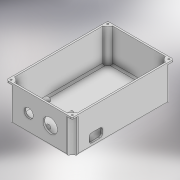
# Autodesk Inventor part: Chasis Raspberry Pi
Saved by Autodesk Inventor 2021.4 (Build 254397000, 397)
## iProperties
Created: 2022-12-12
Part Number: Chasis Raspberry Pi
Material: Genérico
Document SubType Name: Modeling
Designer: crist
Density: 1 g/cm^3
Appearance: Valor por defecto
Mass: 48.8958 g
Surface Area: 495.771 cm^2
Volume: 48.8958 cm^3
Author: crist
Autodesk Inventor part; units mm, degrees
ref_plane "YZ Plane" through (0, 0, 0) normal (1, 0, 0) x (0, 1, 0)
ref_plane "XZ Plane" through (0, 0, 0) normal (0, 1, 0) x (-1, 0, 0)
ref_plane "XY Plane" through (0, 0, 0) normal (0, 0, 1) x (1, 0, 0)
sketch "Boceto1" plane through (0, 0, 0) normal (0, 1, 0) x (-1, 0, 0)
  line L0 (0, 0) -> (78, 0)
  line L1 (78, 0) -> (78, -120)
  line L2 (78, -120) -> (0, -120)
  line L3 (0, -120) -> (0, 0)
  dimension "d0" = 78
  dimension "d1" = 120
  constraints: 8 end point, 2 parallel, 1 horizontal, 1 perpendicular
  measures "d0" distance of L1.end L2.end
  measures "d1" distance of L0.end L1.end
extrude "Extrusión1" add sketch "Boceto1" along normal blind 2
sketch "Boceto2" plane through (0, 2, 0) normal (0, 1, 0) x (1, 0, 0)
  line L0 (0, 120) -> (0, 0) projected
  line L1 (0, 0) -> (-78, 0) projected
  line L2 (-78, 0) -> (-78, 120) projected
  line L3 (-78, 120) -> (0, 120) projected
  line L4 (-76, 118) -> (-76, 2)
  line L5 (-76, 2) -> (-2, 2)
  line L6 (-2, 2) -> (-2, 118)
  line L7 (-2, 118) -> (-76, 118)
  dimension "d4" = 2
  constraints: 8 end point, 3 other
  measures "d4" distance between parallel lines of L2 L4
extrude "Extrusión2" add sketch "Boceto2" along normal blind 40
sketch "Boceto3" plane through (-78, 0, 0) normal (0, 0, 1) x (1, 0, 0)
  line L0 (0, 42) -> (78, 42) projected
  line L1 (78, 42) -> (78, 21)
  line L2 (78, 0) -> (78, 42) projected
  line L3 (78, 21) -> (68, 21)
  line L4 (68, 21) -> (68, 37)
  line L5 (68, 37) -> (36, 37)
  line L6 (36, 37) -> (36, 5)
  line L7 (36, 5) -> (68, 5)
  line L8 (68, 5) -> (68, 21)
  line L9 (36, 37) -> (38, 37)
  line L10 (38, 37) -> (38, 35)
  circle A0 centre (38, 35) radius 1
  line L11 (52, 37) -> (52, 25.2486)
  line L12 (36, 21) -> (50.0571, 21)
  circle A1 centre (66, 35) radius 1
  circle A2 centre (38, 7) radius 1
  circle A3 centre (66, 7) radius 1
  dimension "d7" = 21
  dimension "d8" = 10
  dimension "d9" = 16
  dimension "d10" = 32
  dimension "d11" = 32
  dimension "d12" = 32
  dimension "d13" = 2
  dimension "d14" = 2
  dimension "d15" = 2
  constraints: 22 end point, 5 perpendicular, 4 centre point, 3 midpoint, 3 symmetric about line, 2 point on line, 1 coincident, 1 horizontal, 1 vertical, 3 other
  measures "d7" distance of L0.end L1.end
  measures "d8" distance of L1.end L3.end
  measures "d9" distance of L3.end L4.end
  measures "d10" distance of L4.end L5.end
  measures "d11" distance of L5.end L6.end
  measures "d12" distance of L6.end L7.end
  measures "d13" distance of L5.end L9.end
  measures "d14" distance of L9.end L10.end
  measures "d15" diameter of A0
extrude "Extrusión3" cut sketch "Boceto3" against normal blind 2 contours A0 | A1 | A2 | A3
sketch "Boceto4" plane through (-78, 0, 0) normal (0, 0, 1) x (1, 0, 0)
  line L0 (0, 0) -> (0, 42) projected
  line L1 (0, 42) -> (0, 21)
  line L2 (0, 0) -> (78, 0) projected
  line L3 (0, 21) -> (5, 21)
  line L4 (5, 21) -> (5, 29.01)
  line L5 (5, 29.01) -> (33.28, 29.01)
  line L6 (33.28, 29.01) -> (33.28, 12.99)
  line L7 (33.28, 12.99) -> (5, 12.99)
  line L8 (5, 12.99) -> (5, 21)
  line L9 (5, 21) -> (33.28, 21)
  line L10 (33.28, 21) -> (26.425, 21)
  circle A0 centre (26.425, 21) radius 5.5
  line L11 (33.28, 29.01) -> (31.44, 29.01)
  line L12 (31.44, 29.01) -> (31.44, 27.05)
  circle A1 centre (31.44, 27.05) radius 1
  circle A2 centre (31.44, 14.95) radius 1
  dimension "d18" = 21
  dimension "d19" = 8.01
  dimension "d20" = 28.28
  dimension "d21" = 16.02
  dimension "d22" = 28.28
  dimension "d23" = 6.855
  dimension "d24" = 11
  dimension "d25" = 1.84
  dimension "d26" = 1.96
  dimension "d27" = 2
  dimension "d104" = 5
  constraints: 22 end point, 6 perpendicular, 3 centre point, 2 coincident, 2 point on line, 1 horizontal, 1 midpoint, 1 symmetric about line, 1 other
  measures "d18" distance of L0.end L1.end
  measures "d19" distance of L3.end L4.end
  measures "d20" distance of L4.end L5.end
  measures "d21" distance of L5.end L6.end
  measures "d22" distance of L6.end L7.end
  measures "d23" distance of L9.end L10.end
  measures "d24" diameter of A0
  measures "d25" distance of L5.end L11.end
  measures "d26" distance of L11.end L12.end
  measures "d27" diameter of A1
  measures "d104" distance of L1.end L3.end
extrude "Extrusión4" cut sketch "Boceto4" against normal blind 2 contours A0 L9 | L9 A0 | A1 | A2
fillet "Empalme1" radius 2 16 edges at (-76, 2, -60) (0, 21, 0) (-78, 21, 0) (-39, 0, 0) (0, 0, -60) (-39, 2, -118) (-76, 22, -118) (0, 21, -120) (-2, 22, -118) (-2, 22, -2) (-78, 21, -120) (-2, 2, -60) (-76, 22, -2) (-39, 2, -2) (-39, 0, -120) (-78, 0, -60)
sketch "Boceto5" plane through (-4, 42, -2) normal (0, 0, -1) x (-1, 0, 0)
  line L0 (72, -42) -> (-2, -42) projected
  arc A0 (-4, -40) -> (-2, -42) centre (-2, -40) ccw projected
  line L1 (-4, -40) -> (-4, 0) projected
  line L2 (-4, 0) -> (0, 0) projected
  line L3 (0, 0) -> (70, 0) projected
  line L4 (70, 0) -> (74, 0) projected
  line L5 (74, 0) -> (74, -40) projected
  line L6 (0, 0) -> (0, -38) projected
  line L7 (0, -38) -> (70, -38) projected
  line L8 (70, 0) -> (70, -38) projected
  circle A1 centre (42.56, -27.05) radius 1 projected
  circle A2 centre (42.56, -14.95) radius 1 projected
  circle A3 centre (47.575, -21) radius 5.5 projected
  circle A4 centre (36, -35) radius 1 projected
  circle A5 centre (36, -7) radius 1 projected
  circle A6 centre (8, -35) radius 1 projected
  circle A7 centre (8, -7) radius 1 projected
  circle A8 centre (8, -7) radius 2.5
  circle A9 centre (36, -7) radius 2.5
  circle A10 centre (36, -35) radius 2.5
  circle A11 centre (8, -35) radius 2.5
  arc A12 (72, -42) -> (74, -40) centre (72, -40) ccw projected
  point P0 (-4, -42)
  dimension "d31" = 1.5
  dimension "d32" = 1.5
  dimension "d33" = 1.5
  dimension "d35" = 1.5
  constraints: 4 centre point
  measures "d31" radial gap between concentric circles of A7 A8
  measures "d32" radial gap between concentric circles of A5 A9
  measures "d33" radial gap between concentric circles of A4 A10
  measures "d35" radial gap between concentric circles of A6 A11
extrude "Extrusión5" add sketch "Boceto5" along normal blind 10 contours A8 | A9 | A10 | A11
sketch "Boceto6" plane through (-4, 42, -2) normal (0, 0, -1) x (-1, 0, 0)
  circle A0 centre (8, -7) radius 1 projected
  circle A1 centre (36, -7) radius 1 projected
  line L0 (8, -7) -> (36, -7)
  line L1 (22, -7) -> (22, -21)
  circle A2 centre (22, -21) radius 8.5
  point P0 (-4, -42)
  dimension "d38" = 14
  dimension "d39" = 17
  constraints: 4 end point, 1 centre point, 1 coincident, 1 horizontal, 1 midpoint, 1 vertical
  measures "d38" distance of L1.start L1.end
  measures "d39" diameter of A2
extrude "Extrusión6" cut sketch "Boceto6" against normal blind 2 contours A2
sketch "Boceto7" plane through (-4, 42, -2) normal (0, 0, -1) x (-1, 0, 0)
  circle A0 centre (22, -21) radius 8.5 projected
  circle A1 centre (8, -7) radius 2.5 projected
  circle A2 centre (36, -35) radius 2.5 projected
  circle A3 centre (8, -35) radius 2.5 projected
  circle A4 centre (36, -7) radius 2.5 projected
  line L0 (72, -42) -> (-2, -42) projected
  arc A5 (-4, -40) -> (-2, -42) centre (-2, -40) ccw projected
  line L1 (-4, -40) -> (-4, 0) projected
  line L2 (-4, 0) -> (0, 0) projected
  line L3 (0, 0) -> (70, 0) projected
  line L4 (70, 0) -> (74, 0) projected
  line L5 (74, 0) -> (74, -40) projected
  line L6 (0, 0) -> (0, -38) projected
  line L7 (0, -38) -> (70, -38) projected
  line L8 (70, 0) -> (70, -38) projected
  circle A6 centre (42.56, -27.05) radius 1 projected
  circle A7 centre (42.56, -14.95) radius 1 projected
  circle A8 centre (47.575, -21) radius 5.5 projected
  circle A9 centre (36, -35) radius 1 projected
  circle A10 centre (36, -7) radius 1 projected
  circle A11 centre (8, -35) radius 1 projected
  circle A12 centre (8, -7) radius 1 projected
  arc A13 (44.6263, -16.3572) -> (43.5596, -17.2415) centre (42.56, -14.95) ccw
  arc A14 (43.5596, -24.7585) -> (44.6263, -25.6428) centre (42.56, -27.05) ccw
  arc A15 (72, -42) -> (74, -40) centre (72, -40) ccw projected
  point P0 (-4, -42)
  dimension "d42" = 1.5
  dimension "d43" = 1.5
  constraints: 8 point on circle, 2 centre point
  measures "d42" radial gap between concentric circles of A7 A13
  measures "d43" radial gap between concentric circles of A6 A14
extrude "Extrusión7" add sketch "Boceto7" along normal blind 6 contours A8 A13 | A14 A8
sketch "Boceto8" plane through (-76, 42, 0) normal (0, 0, 1) x (1, 0, 0)
  line L0 (72, -38) -> (2, -38) projected
  line L1 (59.0515, -3.7406) -> (69.5704, -3.7406)
  line L2 (69.5704, -3.7406) -> (69.5704, -38)
  line L3 (69.5704, -38) -> (59.0515, -38)
  line L4 (59.0515, -38) -> (59.0515, -3.7406)
  line L5 (41.825, -36.9742) -> (28.325, -36.9742)
  line L6 (28.325, -36.9742) -> (28.325, -25.9742)
  line L7 (28.325, -25.9742) -> (41.825, -25.9742)
  line L8 (41.825, -25.9742) -> (41.825, -36.9742)
  line L9 (28.325, -16.6878) -> (38.9625, -16.6878)
  line L10 (38.9625, -16.6878) -> (38.9625, -3.7406)
  line L11 (38.9625, -3.7406) -> (28.325, -3.7406)
  line L12 (28.325, -3.7406) -> (28.325, -16.6878)
  dimension "d107" = 11
  dimension "d108" = 13.5
  constraints: 24 end point, 6 parallel, 3 horizontal, 3 perpendicular, 1 point on line
  measures "d107" distance of L7.end L5.start
  measures "d108" distance of L6.end L7.end
extrude "Extrusión8" add sketch "Boceto8" against normal blind 2
sketch "Boceto9" plane through (0, 2, -118) normal (1, 0, 0) x (0, 0, -1)
  line L0 (-85.12, 2.85) -> (-95.02, 2.85)
  line L1 (-98.02, 5.85) -> (-98.02, 10.35)
  line L2 (-95.02, 13.35) -> (-85.12, 13.35)
  line L3 (-82.12, 10.35) -> (-82.12, 5.85)
  arc A0 (-82.12, 10.35) -> (-85.12, 13.35) centre (-85.12, 10.35) ccw
  arc A1 (-85.12, 2.85) -> (-82.12, 5.85) centre (-85.12, 5.85) ccw
  arc A2 (-98.02, 5.85) -> (-95.02, 2.85) centre (-95.02, 5.85) ccw
  arc A3 (-95.02, 13.35) -> (-98.02, 10.35) centre (-95.02, 10.35) ccw
  point P0 (-118, -2)
  point P1 (0, 0)
  point P2 (-98.02, 2.85)
  point P3 (-98.02, 13.35)
  point P4 (-82.12, 13.35)
  dimension "d53" = 10.5
  dimension "d54" = 15.9
  dimension "d55" = 3
  constraints: 8 end point, 8 point on circle, 8 tangent, 6 point on line, 4 centre point, 3 equal radius, 1 horizontal, 1 perpendicular, 1 vertical
  measures "d53" distance of point (-98.02, 2.85) point (-98.02, 13.35)
  measures "d54" distance of point (-98.02, 13.35) point (-82.12, 13.35)
  measures "d55" radius of A0
extrude "Extrusión9" cut sketch "Boceto9" against normal blind 2
sketch "Boceto14" plane through (0, 0, 0) normal (0, -1, 0) x (1, 0, 0)
  arc A0 (-0.8571, -114.0615) -> (-5.9385, -119.1429) centre (0, -120) ccw
  line L0 (0, -120) -> (-2, -118)
  line L1 (-2, -118) -> (-4.2426, -115.7574)
  circle A1 centre (-4.2426, -115.7574) radius 1
  line L2 (-2, -118) -> (-76, -118) projected
  line L3 (-76, -118) -> (-76, -2) projected
  line L4 (-76, -2) -> (-2, -2) projected
  line L5 (-2, -2) -> (-2, -118) projected
  line L6 (-76, -120) -> (-2, -120) projected
  line L7 (-2, -120) -> (-76, -120) projected
  line L8 (-6.9282, -120) -> (-9.9689, -120)
  line L9 (0, -118) -> (0, -2) projected
  line L10 (0, -2) -> (0, -118) projected
  line L11 (0, -113.0718) -> (0, -112.4163)
  arc A2 (-6.9282, -120) -> (-5.9385, -119.1429) centre (-6.9282, -119) ccw
  arc A3 (-0.8571, -114.0615) -> (0, -113.0718) centre (-1, -113.0718) ccw
  arc A4 (-2, -120) -> (0, -118) centre (-2, -118) ccw projected
  line L12 (-39, -120) -> (-39, -100.8346)
  arc A5 (-72.0615, -119.1429) -> (-77.1429, -114.0615) centre (-78, -120) ccw
  line L13 (-78, -120) -> (-76, -118)
  line L14 (-76, -118) -> (-73.7574, -115.7574)
  circle A6 centre (-73.7574, -115.7574) radius 1
  line L15 (-71.0718, -120) -> (-68.0311, -120)
  line L16 (-78, -113.0718) -> (-78, -112.4163)
  arc A7 (-72.0615, -119.1429) -> (-71.0718, -120) centre (-71.0718, -119) ccw
  arc A8 (-78, -113.0718) -> (-77.1429, -114.0615) centre (-77, -113.0718) ccw
  arc A9 (-78, -118) -> (-76, -120) centre (-76, -118) ccw
  line L17 (-78, -2) -> (-78, -118) projected
  line L18 (-78, -118) -> (-78, -2) projected
  line L19 (-78, -60) -> (-55.773, -60)
  line L20 (-2, 0) -> (-76, 0) projected
  line L21 (-78, 0) -> (-76, -2)
  arc A10 (-76, 0) -> (-78, -2) centre (-76, -2) ccw
  circle A11 centre (-73.7574, -4.2426) radius 1
  arc A12 (-77.1429, -5.9385) -> (-72.0615, -0.8571) centre (-78, 0) ccw
  line L22 (-76, -2) -> (-73.7574, -4.2426)
  arc A13 (-71.0718, 0) -> (-72.0615, -0.8571) centre (-71.0718, -1) ccw
  arc A14 (-77.1429, -5.9385) -> (-78, -6.9282) centre (-77, -6.9282) ccw
  line L23 (-78, -6.9282) -> (-78, -7.5837)
  line L24 (-71.0718, 0) -> (-68.0311, 0)
  arc A15 (-5.9385, -0.8571) -> (-0.8571, -5.9385) centre (0, 0) ccw
  line L25 (0, 0) -> (-2, -2)
  line L26 (-2, -2) -> (-4.2426, -4.2426)
  circle A16 centre (-4.2426, -4.2426) radius 1
  line L27 (-6.9282, 0) -> (-9.9689, 0)
  line L28 (0, -6.9282) -> (0, -7.5837)
  arc A17 (-5.9385, -0.8571) -> (-6.9282, 0) centre (-6.9282, -1) ccw
  arc A18 (0, -6.9282) -> (-0.8571, -5.9385) centre (-1, -6.9282) ccw
  arc A19 (0, -2) -> (-2, 0) centre (-2, -2) ccw
  point P0 (0, 0)
  point P1 (-6, -120)
  point P2 (0, -114)
  point P3 (-72, -120)
  point P4 (-78, -114)
  point P5 (-76, -2)
  point P6 (-72, 0)
  point P7 (-78, -6)
  point P8 (-6, 0)
  point P9 (0, -6)
  dimension "d88" = 12
  dimension "d89" = 2
  dimension "d90" = 1
  constraints: 50 symmetric about line, 42 point on circle, 36 end point, 19 centre point, 12 point on line, 4 coincident, 4 tangent, 2 midpoint, 1 equal radius, 1 horizontal, 1 vertical, 15 other
  measures "d88" diameter of A0
  measures "d89" diameter of A1
  measures "d90" radius of A2
extrude "Extrusión10" cut sketch "Boceto14" against normal blind 42 contours A3 L9 A4 L0 L5 A0 | L5 L1 A1 A0 | A1 L1 A0 | A15 A16 L26 L5 | L5 L25 A19 L9 A18 A15 | L2 A0 A1 L1 | L0 A4 L6 A2 A0 L2 | L1 A1 A0 | L26 A16 A15 L4 | L4 A15 A17 L20 A19 L25 | A15 L26 A16 | L26 A15 A16 | A12 A11 L22 L4 | L4 L21 A10 L20 A13 A12 | A5 A7 L6 A9 L13 L2 | L2 L14 A6 A5 | L22 A11 A12 L3 | L3 A12 A14 L17 A10 L21 | A12 L22 A11 | L13 A9 L17 A8 A5 L3 | L3 A5 A6 L14 | A6 L14 A5 | L22 A12 A11 | A6 A5 L14
sketch "Boceto16" plane through (0, 2, 0) normal (0, 1, 0) x (1, 0, 0)
  line L0 (-71.0718, 120) -> (-6.9282, 120) projected
  arc A0 (-5.9385, 119.1429) -> (-6.9282, 120) centre (-6.9282, 119) ccw projected
  arc A1 (-5.9385, 119.1429) -> (-4.4721, 116) centre (0, 120) ccw projected
  arc A2 (-4.4721, 116) -> (-4, 115.5279) centre (0, 120) ccw projected
  arc A3 (-4, 115.5279) -> (-0.8571, 114.0615) centre (0, 120) ccw projected
  arc A4 (0, 113.0718) -> (-0.8571, 114.0615) centre (-1, 113.0718) ccw projected
  line L1 (0, 113.0718) -> (0, 6.9282) projected
  line L2 (-6.9282, 0) -> (-71.0718, 0) projected
  line L3 (-73.5279, 116) -> (-4.4721, 116) projected
  line L4 (-4.4721, 4) -> (-73.5279, 4) projected
  line L5 (-4, 115.5279) -> (-4, 4.4721) projected
  arc A5 (-8, 120) -> (-5.9628, 114.6667) centre (0, 120) ccw
  line L6 (-7.746, 118) -> (-76, 118)
  line L7 (-76, 118) -> (-76, 2)
  line L8 (-76, 2) -> (-2, 2)
  line L9 (-2, 2) -> (-2, 112.254)
  arc A6 (-6.9282, 116) -> (0, 112) centre (0, 120) ccw
  arc A7 (-77.1429, 114.0615) -> (-74, 115.5279) centre (-78, 120) ccw projected
  arc A8 (-74, 115.5279) -> (-73.5279, 116) centre (-78, 120) ccw projected
  arc A9 (-73.5279, 116) -> (-72.0615, 119.1429) centre (-78, 120) ccw projected
  arc A10 (-71.0718, 120) -> (-72.0615, 119.1429) centre (-71.0718, 119) ccw projected
  arc A11 (-77.1429, 114.0615) -> (-78, 113.0718) centre (-77, 113.0718) ccw projected
  line L10 (-78, 6.9282) -> (-78, 113.0718) projected
  arc A12 (-78, 6.9282) -> (-77.1429, 5.9385) centre (-77, 6.9282) ccw projected
  arc A13 (-74, 4.4721) -> (-77.1429, 5.9385) centre (-78, 0) ccw projected
  arc A14 (-73.5279, 4) -> (-74, 4.4721) centre (-78, 0) ccw projected
  arc A15 (-72.0615, 0.8571) -> (-73.5279, 4) centre (-78, 0) ccw projected
  arc A16 (-72.0615, 0.8571) -> (-71.0718, 0) centre (-71.0718, 1) ccw projected
  line L11 (-74, 4.4721) -> (-74, 115.5279) projected
  line L12 (-39, 120) -> (-39, 111.48)
  line L13 (-74, 60) -> (-65.0964, 60)
  arc A17 (-71.0718, 120) -> (-72.0615, 119.1429) centre (-71.0718, 119) ccw
  arc A18 (-73.5279, 116) -> (-72.0615, 119.1429) centre (-78, 120) ccw
  arc A19 (-74, 115.5279) -> (-73.5279, 116) centre (-78, 120) ccw
  arc A20 (-77.1429, 114.0615) -> (-74, 115.5279) centre (-78, 120) ccw
  arc A21 (-77.1429, 114.0615) -> (-78, 113.0718) centre (-77, 113.0718) ccw
  arc A22 (-72.0372, 114.6667) -> (-70, 120) centre (-78, 120) ccw
  arc A23 (-78, 112) -> (-71.0718, 116) centre (-78, 120) ccw
  arc A24 (-74, 4.4721) -> (-77.1429, 5.9385) centre (-78, 0) ccw
  arc A25 (-73.5279, 4) -> (-74, 4.4721) centre (-78, 0) ccw
  arc A26 (-72.0615, 0.8571) -> (-73.5279, 4) centre (-78, 0) ccw
  arc A27 (-72.0615, 0.8571) -> (-71.0718, 0) centre (-71.0718, 1) ccw
  arc A28 (-78, 6.9282) -> (-77.1429, 5.9385) centre (-77, 6.9282) ccw
  arc A29 (-73.5279, 4) -> (-74, 4.4721) centre (-78, 0) ccw
  arc A30 (-74, 4.4721) -> (-77.1429, 5.9385) centre (-78, 0) ccw
  arc A31 (-78, 6.9282) -> (-77.1429, 5.9385) centre (-77, 6.9282) ccw
  arc A32 (-72.0615, 0.8571) -> (-71.0718, 0) centre (-71.0718, 1) ccw
  arc A33 (-70, 0) -> (-72.0372, 5.3333) centre (-78, 0) ccw
  arc A34 (-72.0615, 0.8571) -> (-73.5279, 4) centre (-78, 0) ccw
  arc A35 (-71.0718, 4) -> (-78, 8) centre (-78, 0) ccw
  arc A36 (-0.8571, 5.9385) -> (-4, 4.4721) centre (0, 0) ccw projected
  arc A37 (-4, 4.4721) -> (-4.4721, 4) centre (0, 0) ccw projected
  arc A38 (-4.4721, 4) -> (-5.9385, 0.8571) centre (0, 0) ccw projected
  arc A39 (-6.9282, 0) -> (-5.9385, 0.8571) centre (-6.9282, 1) ccw projected
  arc A40 (-0.8571, 5.9385) -> (0, 6.9282) centre (-1, 6.9282) ccw projected
  arc A41 (-0.8571, 5.9385) -> (0, 6.9282) centre (-1, 6.9282) ccw
  arc A42 (-0.8571, 5.9385) -> (-4, 4.4721) centre (0, 0) ccw
  arc A43 (-4, 4.4721) -> (-4.4721, 4) centre (0, 0) ccw
  arc A44 (-4.4721, 4) -> (-5.9385, 0.8571) centre (0, 0) ccw
  arc A45 (-6.9282, 0) -> (-5.9385, 0.8571) centre (-6.9282, 1) ccw
  arc A46 (-5.9628, 5.3333) -> (-8, 0) centre (0, 0) ccw
  arc A47 (-6.9282, 0) -> (-5.9385, 0.8571) centre (-6.9282, 1) ccw
  arc A48 (-6.9282, 0) -> (-5.9385, 0.8571) centre (-6.9282, 1) ccw
  arc A49 (-4.4721, 4) -> (-5.9385, 0.8571) centre (0, 0) ccw
  arc A50 (-4.4721, 4) -> (-5.9385, 0.8571) centre (0, 0) ccw
  arc A51 (-4, 4.4721) -> (-4.4721, 4) centre (0, 0) ccw
  arc A52 (-4, 4.4721) -> (-4.4721, 4) centre (0, 0) ccw
  arc A53 (-0.8571, 5.9385) -> (-4, 4.4721) centre (0, 0) ccw
  arc A54 (-0.8571, 5.9385) -> (-4, 4.4721) centre (0, 0) ccw
  arc A55 (0, 8) -> (-6.9282, 4) centre (0, 0) ccw
  arc A56 (-0.8571, 5.9385) -> (0, 6.9282) centre (-1, 6.9282) ccw
  arc A57 (-0.8571, 5.9385) -> (0, 6.9282) centre (-1, 6.9282) ccw
  point P0 (0, 0)
  point P1 (-70.254, 118)
  point P2 (-76, 112.254)
  point P3 (-70.254, 2)
  point P4 (-76, 7.746)
  point P5 (-72.0372, 5.3333)
  point P6 (-78, 8)
  point P7 (-78, 112)
  point P8 (-7.746, 2)
  point P9 (-2, 7.746)
  point P10 (-5.9628, 5.3333)
  point P11 (-8, 0)
  point P12 (0, 8)
  dimension "d93" = 2
  constraints: 84 point on circle, 48 symmetric about line, 38 centre point, 12 end point, 3 point on line, 2 midpoint, 1 horizontal, 1 vertical, 37 other
  measures "d93" radial gap between concentric circles of A1 A5
extrude "Extrusión11" add sketch "Boceto16" along normal blind 40 contours L0 A22 L6 A9 A10 | A22 L3 A9 L6 | L0 A0 A1 L3 A5 | A22 A23 L11 A8 L3 | A7 L11 A23 L7 | L7 A23 L10 A11 A7 | L3 A2 L5 A6 A5 | A35 L11 A13 L7 | L7 A13 A12 L10 A35 | A3 A4 L1 A6 L5 | A35 A33 L4 A14 L11 | A55 L9 A36 L5 | L5 A37 L4 A46 A55 | A55 L1 A40 A36 L9 | L4 A33 L8 A15 | L8 A33 L2 A16 A15 | A38 L8 A46 L4 | A38 A39 L2 A46 L8
sketch "Boceto17" plane through (0, 42, 0) normal (0, 1, 0) x (1, 0, 0)
  line L0 (-71.0718, 120) -> (-6.9282, 120) projected
  arc A0 (-5.9385, 119.1429) -> (-6.9282, 120) centre (-6.9282, 119) ccw projected
  arc A1 (-5.9385, 119.1429) -> (-0.8571, 114.0615) centre (0, 120) ccw projected
  arc A2 (0, 113.0718) -> (-0.8571, 114.0615) centre (-1, 113.0718) ccw projected
  line L1 (0, 113.0718) -> (0, 6.9282) projected
  line L2 (-2, 7.746) -> (-2, 112.254) projected
  arc A3 (-7.746, 118) -> (-2, 112.254) centre (0, 120) ccw projected
  line L3 (-7.746, 118) -> (-70.254, 118) projected
  line L4 (-70.254, 2) -> (-7.746, 2) projected
  line L5 (-71.0718, 120) -> (-6.9282, 120) projected
  line L6 (-6.9282, 120) -> (0, 120)
  line L7 (0, 120) -> (0, 113.0718)
  line L8 (0, 6.9282) -> (0, 113.0718) projected
  arc A4 (-72.0615, 0.8571) -> (-77.1429, 5.9385) centre (-78, 0) ccw projected
  arc A5 (-71.0718, 120) -> (-72.0615, 119.1429) centre (-71.0718, 119) ccw projected
  arc A6 (-72.0615, 0.8571) -> (-71.0718, 0) centre (-71.0718, 1) ccw projected
  arc A7 (-77.1429, 114.0615) -> (-72.0615, 119.1429) centre (-78, 120) ccw projected
  arc A8 (-78, 6.9282) -> (-77.1429, 5.9385) centre (-77, 6.9282) ccw projected
  arc A9 (-77.1429, 114.0615) -> (-78, 113.0718) centre (-77, 113.0718) ccw projected
  arc A10 (-76, 112.254) -> (-70.254, 118) centre (-78, 120) ccw projected
  line L9 (-76, 112.254) -> (-76, 7.746) projected
  arc A11 (-70.254, 2) -> (-76, 7.746) centre (-78, 0) ccw projected
  line L10 (-6.9282, 0) -> (-71.0718, 0) projected
  line L11 (-78, 6.9282) -> (-78, 113.0718) projected
  arc A12 (-71.0718, 120) -> (-72.0615, 119.1429) centre (-71.0718, 119) ccw projected
  line L12 (-78, 120) -> (-71.0718, 120)
  line L13 (-78, 0) -> (-71.0718, 0)
  line L14 (-71.0718, 0) -> (-6.9282, 0) projected
  line L15 (-78, 0) -> (-78, 6.9282)
  line L16 (-78, 120) -> (-78, 113.0718)
  line L17 (-78, 113.0718) -> (-78, 6.9282) projected
  arc A13 (-0.8571, 5.9385) -> (0, 6.9282) centre (-1, 6.9282) ccw projected
  arc A14 (-0.8571, 5.9385) -> (-5.9385, 0.8571) centre (0, 0) ccw projected
  arc A15 (-6.9282, 0) -> (-5.9385, 0.8571) centre (-6.9282, 1) ccw projected
  arc A16 (-2, 7.746) -> (-7.746, 2) centre (0, 0) ccw projected
  line L18 (-6.9282, 0) -> (-71.0718, 0) projected
  line L19 (0, 0) -> (-6.9282, 0)
  arc A17 (-0.8571, 5.9385) -> (0, 6.9282) centre (-1, 6.9282) ccw projected
  line L20 (0, 0) -> (0, 6.9282)
  point P0 (0, 0)
  point P1 (-76, 120)
  point P2 (-6.9282, 120)
  constraints: 16 end point, 4 collinear, 3 tangent, 2 horizontal, 1 point on circle, 1 point on line, 1 vertical
extrude "Extrusión12" add sketch "Boceto17" against normal blind 2 contours A5 A7 A9 L16 L12 | L6 L7 A2 A1 A0 | A8 A4 A6 L13 L15 | L20 L19 A15 A14 A13
sketch "Boceto18" plane through (0, 42, 0) normal (0, 1, 0) x (1, 0, 0)
  circle A0 centre (0, 120) radius 4
  line L0 (0, 120) -> (-5.6569, 114.3431)
  arc A1 (-7.746, 118) -> (-2, 112.254) centre (0, 120) ccw projected
  circle A2 centre (-2.8284, 117.1716) radius 1
  arc A3 (-7.746, 118) -> (-2, 112.254) centre (0, 120) ccw
  line L1 (-39, 120) -> (-39, 114.3431)
  line L2 (-76, 60) -> (-65.0745, 60)
  circle A4 centre (-78, 120) radius 4
  line L3 (-78, 120) -> (-72.3431, 114.3431)
  arc A5 (-76, 112.254) -> (-70.254, 118) centre (-78, 120) ccw
  circle A6 centre (-75.1716, 117.1716) radius 1
  arc A7 (-76, 112.254) -> (-70.254, 118) centre (-78, 120) ccw
  circle A8 centre (-78, 0) radius 4
  line L4 (-78, 0) -> (-72.3431, 5.6569)
  arc A9 (-70.254, 2) -> (-76, 7.746) centre (-78, 0) ccw
  circle A10 centre (-75.1716, 2.8284) radius 1
  arc A11 (-70.254, 2) -> (-76, 7.746) centre (-78, 0) ccw
  circle A12 centre (0, 0) radius 4
  line L5 (0, 0) -> (-5.6569, 5.6569)
  arc A13 (-2, 7.746) -> (-7.746, 2) centre (0, 0) ccw
  circle A14 centre (-2.8284, 2.8284) radius 1
  arc A15 (-2, 7.746) -> (-7.746, 2) centre (0, 0) ccw
  dimension "d98" = 8
  dimension "d100" = 2
  constraints: 21 symmetric about line, 18 point on circle, 12 end point, 11 centre point, 4 midpoint, 3 vertical, 2 horizontal, 21 other
  measures "d100" diameter of A2
extrude "Extrusión13" cut sketch "Boceto18" against normal blind 2 contours A2 L0 A0 | A0 L0 A2 | A2 L0 A0 | A0 L0 A2 | A6 L3 A4 | A4 L3 A6 | A6 L3 A4 | A4 L3 A6 | A10 L4 A8 | A8 L4 A10 | A10 L4 A8 | A8 L4 A10 | A14 L5 A12 | A12 L5 A14 | A14 L5 A12 | A12 L5 A14
fillet "Empalme2" radius 2 4 edges at (-78, 41, 0) (-78, 41, -120) (0, 41, -120) (0, 41, 0)
